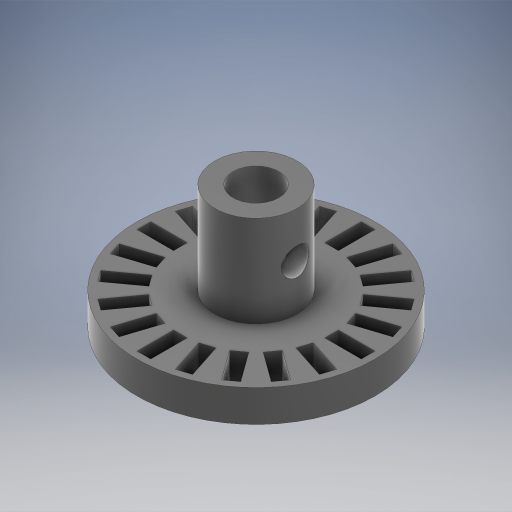
# Autodesk Inventor part: Колесо энкодера
Saved by Autodesk Inventor 2023 (Build 270158000, 158)
## iProperties
Created: 2022-11-09
Part Number: Колесо энкодера
Material: Типовые
Document SubType Name: Modeling
Designer: Admin
Density: 1 g/cm^3
Appearance: По умолчанию
Author: Admin
Autodesk Inventor part; units mm, degrees
ref_plane "XZ Plane" through (0, 0, 0) normal (0, 1, 0) x (-1, 0, 0)
ref_plane "XY Plane" through (0, 0, 0) normal (0, 0, 1) x (1, 0, 0)
sketch "Эскиз1" plane through (0, 0, 0) normal (0, 1, 0) x (-1, 0, 0)
  circle A0 centre (0, 0) radius 2.5
  circle A1 centre (0, 0) radius 7.5
  circle A2 centre (0, 0) radius 13
  line L0 (8.25, 0.75) -> (12.25, 0.75)
  line L1 (12.25, 0.75) -> (12.25, -0.75)
  line L2 (12.25, -0.75) -> (8.25, -0.75)
  line L3 (8.25, -0.75) -> (8.25, 0.75)
  line L4 (8.25, 0.75) -> (12.25, -0.75) construction
  line L5 (12.25, 0.75) -> (8.25, -0.75) construction
  line L6 (13, 0) -> (7.5, 0) construction
  line L7 (7.6145, 3.2627) -> (11.4187, 4.4988)
  line L8 (11.4187, 4.4988) -> (11.8822, 3.0722)
  line L9 (11.8822, 3.0722) -> (8.078, 1.8361)
  line L10 (8.078, 1.8361) -> (7.6145, 3.2627)
  line L11 (7.6145, 3.2627) -> (11.8822, 3.0722) construction
  line L12 (11.4187, 4.4988) -> (8.078, 1.8361) construction
  line L13 (6.2336, 5.456) -> (9.4696, 7.8071)
  line L14 (9.4696, 7.8071) -> (10.3513, 6.5936)
  line L15 (10.3513, 6.5936) -> (7.1152, 4.2425)
  line L16 (7.1152, 4.2425) -> (6.2336, 5.456)
  line L17 (6.2336, 5.456) -> (10.3513, 6.5936) construction
  line L18 (9.4696, 7.8071) -> (7.1152, 4.2425) construction
  line L19 (4.2425, 7.1152) -> (6.5936, 10.3513)
  line L20 (6.5936, 10.3513) -> (7.8071, 9.4696)
  line L21 (7.8071, 9.4696) -> (5.456, 6.2336)
  line L22 (5.456, 6.2336) -> (4.2425, 7.1152)
  line L23 (4.2425, 7.1152) -> (7.8071, 9.4696) construction
  line L24 (6.5936, 10.3513) -> (5.456, 6.2336) construction
  line L25 (1.8361, 8.078) -> (3.0722, 11.8822)
  line L26 (3.0722, 11.8822) -> (4.4988, 11.4187)
  line L27 (4.4988, 11.4187) -> (3.2627, 7.6145)
  line L28 (3.2627, 7.6145) -> (1.8361, 8.078)
  line L29 (1.8361, 8.078) -> (4.4988, 11.4187) construction
  line L30 (3.0722, 11.8822) -> (3.2627, 7.6145) construction
  line L31 (-0.75, 8.25) -> (-0.75, 12.25)
  line L32 (-0.75, 12.25) -> (0.75, 12.25)
  line L33 (0.75, 12.25) -> (0.75, 8.25)
  line L34 (0.75, 8.25) -> (-0.75, 8.25)
  line L35 (-0.75, 8.25) -> (0.75, 12.25) construction
  line L36 (-0.75, 12.25) -> (0.75, 8.25) construction
  line L37 (-3.2627, 7.6145) -> (-4.4988, 11.4187)
  line L38 (-4.4988, 11.4187) -> (-3.0722, 11.8822)
  line L39 (-3.0722, 11.8822) -> (-1.8361, 8.078)
  line L40 (-1.8361, 8.078) -> (-3.2627, 7.6145)
  line L41 (-3.2627, 7.6145) -> (-3.0722, 11.8822) construction
  line L42 (-4.4988, 11.4187) -> (-1.8361, 8.078) construction
  line L43 (-5.456, 6.2336) -> (-7.8071, 9.4696)
  line L44 (-7.8071, 9.4696) -> (-6.5936, 10.3513)
  line L45 (-6.5936, 10.3513) -> (-4.2425, 7.1152)
  line L46 (-4.2425, 7.1152) -> (-5.456, 6.2336)
  line L47 (-5.456, 6.2336) -> (-6.5936, 10.3513) construction
  line L48 (-7.8071, 9.4696) -> (-4.2425, 7.1152) construction
  line L49 (-7.1152, 4.2425) -> (-10.3513, 6.5936)
  line L50 (-10.3513, 6.5936) -> (-9.4696, 7.8071)
  line L51 (-9.4696, 7.8071) -> (-6.2336, 5.456)
  line L52 (-6.2336, 5.456) -> (-7.1152, 4.2425)
  line L53 (-7.1152, 4.2425) -> (-9.4696, 7.8071) construction
  line L54 (-10.3513, 6.5936) -> (-6.2336, 5.456) construction
  line L55 (-8.078, 1.8361) -> (-11.8822, 3.0722)
  line L56 (-11.8822, 3.0722) -> (-11.4187, 4.4988)
  line L57 (-11.4187, 4.4988) -> (-7.6145, 3.2627)
  line L58 (-7.6145, 3.2627) -> (-8.078, 1.8361)
  line L59 (-8.078, 1.8361) -> (-11.4187, 4.4988) construction
  line L60 (-11.8822, 3.0722) -> (-7.6145, 3.2627) construction
  line L61 (-8.25, -0.75) -> (-12.25, -0.75)
  line L62 (-12.25, -0.75) -> (-12.25, 0.75)
  line L63 (-12.25, 0.75) -> (-8.25, 0.75)
  line L64 (-8.25, 0.75) -> (-8.25, -0.75)
  line L65 (-8.25, -0.75) -> (-12.25, 0.75) construction
  line L66 (-12.25, -0.75) -> (-8.25, 0.75) construction
  line L67 (-7.6145, -3.2627) -> (-11.4187, -4.4988)
  line L68 (-11.4187, -4.4988) -> (-11.8822, -3.0722)
  line L69 (-11.8822, -3.0722) -> (-8.078, -1.8361)
  line L70 (-8.078, -1.8361) -> (-7.6145, -3.2627)
  line L71 (-7.6145, -3.2627) -> (-11.8822, -3.0722) construction
  line L72 (-11.4187, -4.4988) -> (-8.078, -1.8361) construction
  line L73 (-6.2336, -5.456) -> (-9.4696, -7.8071)
  line L74 (-9.4696, -7.8071) -> (-10.3513, -6.5936)
  line L75 (-10.3513, -6.5936) -> (-7.1152, -4.2425)
  line L76 (-7.1152, -4.2425) -> (-6.2336, -5.456)
  line L77 (-6.2336, -5.456) -> (-10.3513, -6.5936) construction
  line L78 (-9.4696, -7.8071) -> (-7.1152, -4.2425) construction
  line L79 (-4.2425, -7.1152) -> (-6.5936, -10.3513)
  line L80 (-6.5936, -10.3513) -> (-7.8071, -9.4696)
  line L81 (-7.8071, -9.4696) -> (-5.456, -6.2336)
  line L82 (-5.456, -6.2336) -> (-4.2425, -7.1152)
  line L83 (-4.2425, -7.1152) -> (-7.8071, -9.4696) construction
  line L84 (-6.5936, -10.3513) -> (-5.456, -6.2336) construction
  line L85 (-1.8361, -8.078) -> (-3.0722, -11.8822)
  line L86 (-3.0722, -11.8822) -> (-4.4988, -11.4187)
  line L87 (-4.4988, -11.4187) -> (-3.2627, -7.6145)
  line L88 (-3.2627, -7.6145) -> (-1.8361, -8.078)
  line L89 (-1.8361, -8.078) -> (-4.4988, -11.4187) construction
  line L90 (-3.0722, -11.8822) -> (-3.2627, -7.6145) construction
  line L91 (0.75, -8.25) -> (0.75, -12.25)
  line L92 (0.75, -12.25) -> (-0.75, -12.25)
  line L93 (-0.75, -12.25) -> (-0.75, -8.25)
  line L94 (-0.75, -8.25) -> (0.75, -8.25)
  line L95 (0.75, -8.25) -> (-0.75, -12.25) construction
  line L96 (0.75, -12.25) -> (-0.75, -8.25) construction
  line L97 (3.2627, -7.6145) -> (4.4988, -11.4187)
  line L98 (4.4988, -11.4187) -> (3.0722, -11.8822)
  line L99 (3.0722, -11.8822) -> (1.8361, -8.078)
  line L100 (1.8361, -8.078) -> (3.2627, -7.6145)
  line L101 (3.2627, -7.6145) -> (3.0722, -11.8822) construction
  line L102 (4.4988, -11.4187) -> (1.8361, -8.078) construction
  line L103 (5.456, -6.2336) -> (7.8071, -9.4696)
  line L104 (7.8071, -9.4696) -> (6.5936, -10.3513)
  line L105 (6.5936, -10.3513) -> (4.2425, -7.1152)
  line L106 (4.2425, -7.1152) -> (5.456, -6.2336)
  line L107 (5.456, -6.2336) -> (6.5936, -10.3513) construction
  line L108 (7.8071, -9.4696) -> (4.2425, -7.1152) construction
  line L109 (7.1152, -4.2425) -> (10.3513, -6.5936)
  line L110 (10.3513, -6.5936) -> (9.4696, -7.8071)
  line L111 (9.4696, -7.8071) -> (6.2336, -5.456)
  line L112 (6.2336, -5.456) -> (7.1152, -4.2425)
  line L113 (7.1152, -4.2425) -> (9.4696, -7.8071) construction
  line L114 (10.3513, -6.5936) -> (6.2336, -5.456) construction
  line L115 (8.078, -1.8361) -> (11.8822, -3.0722)
  line L116 (11.8822, -3.0722) -> (11.4187, -4.4988)
  line L117 (11.4187, -4.4988) -> (7.6145, -3.2627)
  line L118 (7.6145, -3.2627) -> (8.078, -1.8361)
  line L119 (8.078, -1.8361) -> (11.4187, -4.4988) construction
  line L120 (11.8822, -3.0722) -> (7.6145, -3.2627) construction
  circle A3 centre (0, 0) radius 10.25 construction
  point P0 (10.25, 0)
  point P1 (10.25, 0)
  point P2 (10.25, 0)
  point P3 (9.7483, 3.1674)
  point P4 (9.7483, 3.1674)
  point P5 (9.7483, 3.1674)
  point P6 (8.2924, 6.0248)
  point P7 (8.2924, 6.0248)
  point P8 (8.2924, 6.0248)
  point P9 (6.0248, 8.2924)
  point P10 (6.0248, 8.2924)
  point P11 (6.0248, 8.2924)
  point P12 (3.1674, 9.7483)
  point P13 (3.1674, 9.7483)
  point P14 (3.1674, 9.7483)
  point P15 (0, 10.25)
  point P16 (0, 10.25)
  point P17 (0, 10.25)
  point P18 (-3.1674, 9.7483)
  point P19 (-3.1674, 9.7483)
  point P20 (-3.1674, 9.7483)
  point P21 (-6.0248, 8.2924)
  point P22 (-6.0248, 8.2924)
  point P23 (-6.0248, 8.2924)
  point P24 (-8.2924, 6.0248)
  point P25 (-8.2924, 6.0248)
  point P26 (-8.2924, 6.0248)
  point P27 (-9.7483, 3.1674)
  point P28 (-9.7483, 3.1674)
  point P29 (-9.7483, 3.1674)
  point P30 (-10.25, 0)
  point P31 (-10.25, 0)
  point P32 (-10.25, 0)
  point P33 (-9.7483, -3.1674)
  point P34 (-9.7483, -3.1674)
  point P35 (-9.7483, -3.1674)
  point P36 (-8.2924, -6.0248)
  point P37 (-8.2924, -6.0248)
  point P38 (-8.2924, -6.0248)
  point P39 (-6.0248, -8.2924)
  point P40 (-6.0248, -8.2924)
  point P41 (-6.0248, -8.2924)
  point P42 (-3.1674, -9.7483)
  point P43 (-3.1674, -9.7483)
  point P44 (-3.1674, -9.7483)
  point P45 (0, -10.25)
  point P46 (0, -10.25)
  point P47 (0, -10.25)
  point P48 (3.1674, -9.7483)
  point P49 (3.1674, -9.7483)
  point P50 (3.1674, -9.7483)
  point P51 (6.0248, -8.2924)
  point P52 (6.0248, -8.2924)
  point P53 (6.0248, -8.2924)
  point P54 (8.2924, -6.0248)
  point P55 (8.2924, -6.0248)
  point P56 (8.2924, -6.0248)
  point P57 (9.7483, -3.1674)
  point P58 (9.7483, -3.1674)
  point P59 (9.7483, -3.1674)
  dimension "d1" = 15
  dimension "d2" = 26
  dimension "d0" = 5
  dimension "d3" = 4
  dimension "d4" = 1.5
  dimension "d7" = 360
  constraints: 242 end point, 43 midpoint, 4 coincident, 3 horizontal alignment, 2 horizontal, 2 parallel, 1 centre point, 1 perpendicular, 1 vertical alignment, 267 other
  measures "d0" diameter of A0
  measures "d3" distance of L1.end L2.end
  measures "d4" distance of L0.end L1.end
extrude "Выдавливание1" add sketch "Эскиз1" along normal blind 2.5 contours A1 | A2
sketch "Эскиз2" plane through (0, 2.5, 0) normal (0, 1, 0) x (1, 0, 0)
  circle A0 centre (0, 0) radius 13 projected
  circle A1 centre (0, 0) radius 2.5 projected
  line L0 (-8.078, 1.8361) -> (-11.8822, 3.0722) projected
  line L1 (-11.8822, 3.0722) -> (-11.4187, 4.4988) projected
  line L2 (-11.4187, 4.4988) -> (-7.6145, 3.2627) projected
  line L3 (-7.6145, 3.2627) -> (-8.078, 1.8361) projected
  line L4 (-7.1152, 4.2425) -> (-10.3513, 6.5936) projected
  line L5 (-10.3513, 6.5936) -> (-9.4696, 7.8071) projected
  line L6 (-9.4696, 7.8071) -> (-6.2336, 5.456) projected
  line L7 (-6.2336, 5.456) -> (-7.1152, 4.2425) projected
  line L8 (-5.456, 6.2336) -> (-7.8071, 9.4696) projected
  line L9 (-7.8071, 9.4696) -> (-6.5936, 10.3513) projected
  line L10 (-6.5936, 10.3513) -> (-4.2425, 7.1152) projected
  line L11 (-4.2425, 7.1152) -> (-5.456, 6.2336) projected
  line L12 (-3.2627, 7.6145) -> (-4.4988, 11.4187) projected
  line L13 (-4.4988, 11.4187) -> (-3.0722, 11.8822) projected
  line L14 (-3.0722, 11.8822) -> (-1.8361, 8.078) projected
  line L15 (-1.8361, 8.078) -> (-3.2627, 7.6145) projected
  line L16 (-0.75, 8.25) -> (-0.75, 12.25) projected
  line L17 (-0.75, 12.25) -> (0.75, 12.25) projected
  line L18 (0.75, 12.25) -> (0.75, 8.25) projected
  line L19 (0.75, 8.25) -> (-0.75, 8.25) projected
  line L20 (1.8361, 8.078) -> (3.0722, 11.8822) projected
  line L21 (3.0722, 11.8822) -> (4.4988, 11.4187) projected
  line L22 (4.4988, 11.4187) -> (3.2627, 7.6145) projected
  line L23 (3.2627, 7.6145) -> (1.8361, 8.078) projected
  line L24 (4.2425, 7.1152) -> (6.5936, 10.3513) projected
  line L25 (6.5936, 10.3513) -> (7.8071, 9.4696) projected
  line L26 (7.8071, 9.4696) -> (5.456, 6.2336) projected
  line L27 (5.456, 6.2336) -> (4.2425, 7.1152) projected
  line L28 (6.2336, 5.456) -> (9.4696, 7.8071) projected
  line L29 (9.4696, 7.8071) -> (10.3513, 6.5936) projected
  line L30 (10.3513, 6.5936) -> (7.1152, 4.2425) projected
  line L31 (7.1152, 4.2425) -> (6.2336, 5.456) projected
  line L32 (7.6145, 3.2627) -> (11.4187, 4.4988) projected
  line L33 (11.4187, 4.4988) -> (11.8822, 3.0722) projected
  line L34 (11.8822, 3.0722) -> (8.078, 1.8361) projected
  line L35 (8.078, 1.8361) -> (7.6145, 3.2627) projected
  line L36 (8.25, 0.75) -> (12.25, 0.75) projected
  line L37 (12.25, 0.75) -> (12.25, -0.75) projected
  line L38 (12.25, -0.75) -> (8.25, -0.75) projected
  line L39 (8.25, -0.75) -> (8.25, 0.75) projected
  line L40 (8.078, -1.8361) -> (11.8822, -3.0722) projected
  line L41 (11.8822, -3.0722) -> (11.4187, -4.4988) projected
  line L42 (11.4187, -4.4988) -> (7.6145, -3.2627) projected
  line L43 (7.6145, -3.2627) -> (8.078, -1.8361) projected
  line L44 (7.1152, -4.2425) -> (10.3513, -6.5936) projected
  line L45 (10.3513, -6.5936) -> (9.4696, -7.8071) projected
  line L46 (9.4696, -7.8071) -> (6.2336, -5.456) projected
  line L47 (6.2336, -5.456) -> (7.1152, -4.2425) projected
  line L48 (5.456, -6.2336) -> (7.8071, -9.4696) projected
  line L49 (7.8071, -9.4696) -> (6.5936, -10.3513) projected
  line L50 (6.5936, -10.3513) -> (4.2425, -7.1152) projected
  line L51 (4.2425, -7.1152) -> (5.456, -6.2336) projected
  line L52 (3.2627, -7.6145) -> (4.4988, -11.4187) projected
  line L53 (4.4988, -11.4187) -> (3.0722, -11.8822) projected
  line L54 (3.0722, -11.8822) -> (1.8361, -8.078) projected
  line L55 (1.8361, -8.078) -> (3.2627, -7.6145) projected
  line L56 (0.75, -8.25) -> (0.75, -12.25) projected
  line L57 (0.75, -12.25) -> (-0.75, -12.25) projected
  line L58 (-0.75, -12.25) -> (-0.75, -8.25) projected
  line L59 (-0.75, -8.25) -> (0.75, -8.25) projected
  line L60 (-1.8361, -8.078) -> (-3.0722, -11.8822) projected
  line L61 (-3.0722, -11.8822) -> (-4.4988, -11.4187) projected
  line L62 (-4.4988, -11.4187) -> (-3.2627, -7.6145) projected
  line L63 (-3.2627, -7.6145) -> (-1.8361, -8.078) projected
  line L64 (-4.2425, -7.1152) -> (-6.5936, -10.3513) projected
  line L65 (-6.5936, -10.3513) -> (-7.8071, -9.4696) projected
  line L66 (-7.8071, -9.4696) -> (-5.456, -6.2336) projected
  line L67 (-5.456, -6.2336) -> (-4.2425, -7.1152) projected
  line L68 (-6.2336, -5.456) -> (-9.4696, -7.8071) projected
  line L69 (-9.4696, -7.8071) -> (-10.3513, -6.5936) projected
  line L70 (-10.3513, -6.5936) -> (-7.1152, -4.2425) projected
  line L71 (-7.1152, -4.2425) -> (-6.2336, -5.456) projected
  line L72 (-7.6145, -3.2627) -> (-11.4187, -4.4988) projected
  line L73 (-11.4187, -4.4988) -> (-11.8822, -3.0722) projected
  line L74 (-11.8822, -3.0722) -> (-8.078, -1.8361) projected
  line L75 (-8.078, -1.8361) -> (-7.6145, -3.2627) projected
  line L76 (-8.25, -0.75) -> (-12.25, -0.75) projected
  line L77 (-12.25, -0.75) -> (-12.25, 0.75) projected
  line L78 (-12.25, 0.75) -> (-8.25, 0.75) projected
  line L79 (-8.25, 0.75) -> (-8.25, -0.75) projected
extrude "Выдавливание2" add sketch "Эскиз2" along normal blind 1
sketch "Эскиз4" plane through (0, 3.5, 0) normal (0, 1, 0) x (1, 0, 0)
  circle A0 centre (0, 0) radius 4.5
  circle A1 centre (0, 0) radius 2.5 projected
  dimension "d16" = 2
  constraints: 1 centre point, 1 coincident
  measures "d16" radial gap between concentric circles of A1 A0
extrude "Выдавливание4" add sketch "Эскиз4" along normal blind 10
ref_plane "РабПлоскость1" through (13, 0, 0) normal (1, 0, 0) x (0, 1, 0)
sketch "Эскиз5" plane through (13, 0, 0) normal (1, 0, 0) x (0, 1, 0)
  circle A0 centre (8.5, 0) radius 1.5
  line L0 (3.5, -4.5) -> (13.5, -4.5) projected
  point P0 (0, 0)
  point P1 (8.5, -4.5)
  dimension "d19" = 3
  constraints: 1 centre point, 1 horizontal alignment, 1 midpoint, 1 vertical alignment
  measures "d19" diameter of A0
extrude "Выдавливание5" cut sketch "Эскиз5" against normal up to surface round surface about axis through (0, 0, 0) along (0, 1, 0) radius 2.5 far side no
